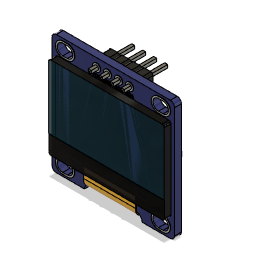
Tela OLed 128x64 v15 (Autodesk Fusion 360 design; units mm, degrees)
Autodesk Fusion 360 part; units mm, degrees
(part 1 of 2)
sketch "Sketch1" plane through (0, 0, 0) normal (0, 0, 1) x (1, 0, 0)
  line L0 (13.34, -9.6) -> (-13.34, -9.6)
  line L1 (-13.34, -9.6) -> (-13.34, 9.6)
  line L2 (-13.34, 9.6) -> (13.34, 9.6)
  line L3 (13.34, 9.6) -> (13.34, -9.6)
  line L4 (13.34, -9.6) -> (-13.34, 9.6) construction
  line L5 (-13.34, -9.6) -> (13.34, 9.6) construction
  dimension "d1" = 26.68
  dimension "d2" = 19.2
  constraint horizontal L0
  constraint perpendicular L0 L1
  constraint parallel L0 L2
  constraint parallel L1 L3
  constraint coincident L4 origin
  constraint coincident L5 origin
  measures "d1" distance of L1.end L2.end
  measures "d2" distance of L0.end L1.end
extrude "Extrude1" add sketch "Sketch1" along normal blind 1.5 makes body 1
sketch "Sketch2" plane through (0, 0, 1.5) normal (0, 0, 1) x (1, 0, 0)
  line L0 (13.34, 9.6) -> (-13.34, 9.6)
  line L1 (-13.34, 9.6) -> (-13.34, -9.6)
  line L2 (-13.34, -9.6) -> (13.34, -9.6)
  line L3 (13.34, -9.6) -> (13.34, 9.6)
  line L4 (-13.34, 9.6) -> (13.34, 9.6)
  line L5 (13.34, 9.6) -> (13.34, -5.4)
  line L6 (13.34, -5.4) -> (-13.34, -5.4)
  line L7 (-13.34, -5.4) -> (-13.34, 9.6)
  dimension "d5" = 15
  constraint horizontal L4
  constraint vertical L5
  constraint horizontal L6
  constraint vertical L7
  constraint coincident L3 L5.end
  constraint coincident L0.end L1.start
  measures "d5" distance of L0.end L6.end
extrude "Extrude2" add sketch "Sketch2" along normal blind 0.1 contours L0 L1 L3 L4 L5 L6 L7 bodies 1
copy_body "Body->Comp1" bodies 1 removing the originals makes body 2 in component "Pantalla"
sketch "Sketch1 (2)" plane through (0, 0, 0) normal (0, 0, -1) x (-1, 0, 0) in component "Base PCB"
  line L0 (13.34, 9.6) -> (-13.34, 9.6) construction
  line L1 (-13.34, 9.6) -> (-13.34, -9.6) construction
  line L2 (-13.34, -9.6) -> (13.34, -9.6) construction
  line L3 (13.34, -9.6) -> (13.34, 9.6) construction
  line L4 (-14.15, 14.25) -> (14.15, 14.25)
  line L5 (14.15, 14.25) -> (14.15, -13.4)
  line L6 (14.15, -13.4) -> (-14.15, -13.4)
  line L7 (-14.15, -13.4) -> (-14.15, 14.25)
  dimension "d8" = 27.65
  dimension "d9" = 28.3
  dimension "d10" = 3.8
  dimension "d11" = 0.81
  constraint horizontal L4
  constraint vertical L5
  constraint horizontal L6
  constraint vertical L7
  measures "d8" distance of L4.end L5.end
  measures "d9" distance of L4.start L4.end
  measures "d10" distance of L2 L6
  measures "d11" distance of L1 L7
extrude "Extrude1'" add sketch "Sketch1 (2)" along normal blind 1.6 separate body makes body 3 in component "Base PCB"
sketch "Sketch2 (2)" plane through (0, 0, 0) normal (0, 0, 1) x (1, 0, 0) in component "Base PCB"
  line L0 (-14.15, -13.4) -> (14.15, -13.4)
  line L1 (14.15, -13.4) -> (14.15, 14.25)
  line L2 (14.15, 14.25) -> (-14.15, 14.25)
  line L3 (-14.15, 14.25) -> (-14.15, -13.4)
  line L4 (-11.575, 10.9) -> (-10.525, 10.9) construction
  arc A0 (-10.525, 10.9) -> (-10.525, 13.25) centre (-10.525, 12.075) ccw construction
  line L5 (-10.525, 13.25) -> (-11.575, 13.25) construction
  arc A1 (-11.575, 13.25) -> (-11.575, 10.9) centre (-11.575, 12.075) ccw construction
  line L6 (-11.575, 12.075) -> (-10.525, 12.075) construction
  line L7 (0, 14.25) -> (0, 0) construction
  line L8 (0, 0) -> (14.15, 0) construction
  arc A2 (-10.525, 10.8) -> (-10.525, 13.35) centre (-10.525, 12.075) ccw
  line L9 (-10.525, 13.35) -> (-11.575, 13.35)
  arc A3 (-11.575, 13.35) -> (-11.575, 10.8) centre (-11.575, 12.075) ccw
  line L10 (-11.575, 10.8) -> (-10.525, 10.8)
  arc A4 (10.525, 13.35) -> (10.525, 10.8) centre (10.525, 12.075) ccw
  line L11 (10.525, 13.35) -> (11.575, 13.35)
  arc A5 (11.575, 10.8) -> (11.575, 13.35) centre (11.575, 12.075) ccw
  line L12 (11.575, 10.8) -> (10.525, 10.8)
  line L13 (-14.15, 0.425) -> (-23.1438, 0.425) construction
  line L14 (-10.525, -12.5) -> (-11.575, -12.5)
  arc A6 (-11.575, -9.95) -> (-11.575, -12.5) centre (-11.575, -11.225) ccw
  line L15 (-11.575, -9.95) -> (-10.525, -9.95)
  arc A7 (-10.525, -12.5) -> (-10.525, -9.95) centre (-10.525, -11.225) ccw
  line L16 (10.525, -12.5) -> (11.575, -12.5)
  arc A8 (10.525, -9.95) -> (10.525, -12.5) centre (10.525, -11.225) ccw
  line L17 (11.575, -9.95) -> (10.525, -9.95)
  arc A9 (11.575, -12.5) -> (11.575, -9.95) centre (11.575, -11.225) ccw
  point P0 (-12.75, 12.075)
  dimension "d14" = 1.175
  dimension "d15" = 1.05
  dimension "d16" = 1
  dimension "d17" = 1.4
  dimension "d18" = 0.1
  constraint tangent L4 A0
  constraint tangent A0 L5
  constraint parallel L4 L5
  constraint tangent L5 A1
  constraint tangent L4 A1
  constraint horizontal L6
  constraint midpoint A1 P0
  constraint midpoint L2 L7.start
  constraint coincident L7.end L8.start
  constraint coincident L1 L8.end
  constraint perpendicular L1 L8
  constraint symmetric L7 A2.end A4.start
  constraint symmetric L7 A2.start A4.end
  constraint symmetric L7 A2 A4
  constraint symmetric L7 L9.end L11.end
  constraint symmetric L7 A3.end A5.start
  constraint symmetric L7 A3 A5
  constraint midpoint L3 L13.start
  constraint perpendicular L3 L13
  constraint symmetric A2.end L13 L14.start
  constraint symmetric A2.start L13 L15.end
  constraint symmetric A2 L13 A7
  constraint symmetric L9.end L13 L14.end
  constraint symmetric A3.end L13 A6.start
  constraint symmetric A3 L13 A6
  constraint symmetric A4.end L13 A8.start
  constraint symmetric A4.start L13 L16.start
  constraint symmetric A4 L13 A8
  constraint symmetric L11.end L13 L16.end
  constraint symmetric A5.start L13 L17.start
  constraint symmetric A5 L13 A9
  measures "d14" radius of A1
  measures "d15" distance of A1.centre A0.centre
  measures "d16" distance of L2 L5
  measures "d17" distance of L3 P0
extrude "Extrude2'" cut sketch "Sketch2 (2)" against normal through all contours A2 L9 A3 L10 | A4 L11 A5 L12 | L14 A6 L15 A7 | L16 A8 L17 A9 bodies 3 in component "Base PCB"
fillet "Fillet1" radius 1 4 edges at (-14.15, 14.25, -0.8) (14.15, 14.25, -0.8) (-14.15, -13.4, -0.8) (14.15, -13.4, -0.8) on bodies 3 in component "Base PCB"
sketch "Sketch3" plane through (0, 0, 0) normal (0, 0, 1) x (1, 0, 0) in component "Base PCB"
  line L0 (10.525, 13.35) -> (11.575, 13.35)
  arc A0 (11.575, 10.8) -> (11.575, 13.35) centre (11.575, 12.075) ccw
  line L1 (11.575, 10.8) -> (10.525, 10.8)
  arc A1 (10.525, 13.35) -> (10.525, 10.8) centre (10.525, 12.075) ccw
  line L2 (-11.575, -9.95) -> (-10.525, -9.95)
  arc A2 (-10.525, -12.5) -> (-10.525, -9.95) centre (-10.525, -11.225) ccw
  line L3 (-10.525, -12.5) -> (-11.575, -12.5)
  arc A3 (-11.575, -9.95) -> (-11.575, -12.5) centre (-11.575, -11.225) ccw
  arc A4 (-11.575, 13.35) -> (-11.575, 10.8) centre (-11.575, 12.075) ccw
  line L4 (-11.575, 13.35) -> (-10.525, 13.35)
  arc A5 (-10.525, 10.8) -> (-10.525, 13.35) centre (-10.525, 12.075) ccw
  line L5 (-10.525, 10.8) -> (-11.575, 10.8)
  line L6 (11.575, -12.5) -> (10.525, -12.5)
  arc A6 (10.525, -9.95) -> (10.525, -12.5) centre (10.525, -11.225) ccw
  line L7 (10.525, -9.95) -> (11.575, -9.95)
  arc A7 (11.575, -12.5) -> (11.575, -9.95) centre (11.575, -11.225) ccw
  arc A8 (13.15, -13.4) -> (14.15, -12.4) centre (13.15, -12.4) ccw
  line L8 (14.15, -12.4) -> (14.15, 13.25)
  arc A9 (14.15, 13.25) -> (13.15, 14.25) centre (13.15, 13.25) ccw
  line L9 (13.15, 14.25) -> (-13.15, 14.25)
  arc A10 (-13.15, 14.25) -> (-14.15, 13.25) centre (-13.15, 13.25) ccw
  line L10 (-14.15, 13.25) -> (-14.15, -12.4)
  arc A11 (-14.15, -12.4) -> (-13.15, -13.4) centre (-13.15, -12.4) ccw
  line L11 (-13.15, -13.4) -> (13.15, -13.4)
  line L12 (-5.5683, 12.35) -> (5.9249, 12.35) construction
  circle A12 centre (-1.27, 12.35) radius 0.5
  circle A13 centre (-1.27, 12.35) radius 0.9
  line L13 (0, 14.25) -> (0, 16.388) construction
  circle A14 centre (-3.81, 12.35) radius 0.5
  circle A15 centre (-3.81, 12.35) radius 0.9
  circle A16 centre (3.81, 12.35) radius 0.9
  circle A17 centre (3.81, 12.35) radius 0.5
  circle A18 centre (1.27, 12.35) radius 0.9
  circle A19 centre (1.27, 12.35) radius 0.5
  dimension "d22" = 1.9
  dimension "d23" = 1
  dimension "d24" = 0.4
  dimension "d25" = 1.27
  dimension "d26" = 2.54
  constraint parallel L5 L12
  constraint coincident L12 A12.centre
  constraint midpoint L9 L13.start
  constraint perpendicular L9 L13
  constraint coincident L12 A14.centre
  constraint concentric A14 A15
  constraint equal A12 A14
  constraint equal A13 A15
  constraint symmetric A12 L13 A19
  constraint symmetric A13 L13 A18
  constraint symmetric L13 A14 A17
  constraint symmetric L13 A15 A16
  measures "d22" distance of L9 L12
  measures "d23" diameter of A12
  measures "d25" distance of A12.centre L13
  measures "d26" distance of A12.centre A14.centre
extrude "Extrude3" cut sketch "Sketch3" against normal through all contours A12 | A14 | A17 | A19 bodies 3 in component "Base PCB"
extrude "Extrude4" add sketch "Sketch3" along normal blind 0.1 contours A13 | A15 | A16 | A18 bodies 3 in component "Base PCB"
sketch "Sketch4" plane through (0, 0, 0) normal (0, 0, 1) x (1, 0, 0) in component "Base PCB"
  circle A0 centre (3.81, 12.35) radius 0.9
  circle A1 centre (-3.81, 12.35) radius 0.9
  circle A2 centre (1.27, 12.35) radius 0.9
  circle A3 centre (-1.27, 12.35) radius 0.9
  line L0 (10.525, 13.35) -> (11.575, 13.35)
  arc A4 (11.575, 10.8) -> (11.575, 13.35) centre (11.575, 12.075) ccw
  line L1 (11.575, 10.8) -> (10.525, 10.8)
  arc A5 (10.525, 13.35) -> (10.525, 10.8) centre (10.525, 12.075) ccw
  line L2 (-11.575, -9.95) -> (-10.525, -9.95)
  arc A6 (-10.525, -12.5) -> (-10.525, -9.95) centre (-10.525, -11.225) ccw
  line L3 (-10.525, -12.5) -> (-11.575, -12.5)
  arc A7 (-11.575, -9.95) -> (-11.575, -12.5) centre (-11.575, -11.225) ccw
  arc A8 (-11.575, 13.35) -> (-11.575, 10.8) centre (-11.575, 12.075) ccw
  line L4 (-11.575, 13.35) -> (-10.525, 13.35)
  arc A9 (-10.525, 10.8) -> (-10.525, 13.35) centre (-10.525, 12.075) ccw
  line L5 (-10.525, 10.8) -> (-11.575, 10.8)
  line L6 (11.575, -12.5) -> (10.525, -12.5)
  arc A10 (10.525, -9.95) -> (10.525, -12.5) centre (10.525, -11.225) ccw
  line L7 (10.525, -9.95) -> (11.575, -9.95)
  arc A11 (11.575, -12.5) -> (11.575, -9.95) centre (11.575, -11.225) ccw
  arc A12 (13.15, -13.4) -> (14.15, -12.4) centre (13.15, -12.4) ccw
  line L8 (14.15, -12.4) -> (14.15, 13.25)
  arc A13 (14.15, 13.25) -> (13.15, 14.25) centre (13.15, 13.25) ccw
  line L9 (13.15, 14.25) -> (-13.15, 14.25)
  arc A14 (-13.15, 14.25) -> (-14.15, 13.25) centre (-13.15, 13.25) ccw
  line L10 (-14.15, 13.25) -> (-14.15, -12.4)
  arc A15 (-14.15, -12.4) -> (-13.15, -13.4) centre (-13.15, -12.4) ccw
  line L11 (-13.15, -13.4) -> (13.15, -13.4)
  arc A16 (-10.525, 10.4) -> (-10.525, 13.75) centre (-10.525, 12.075) ccw
  line L12 (-11.575, 13.75) -> (-10.525, 13.75)
  arc A17 (-11.575, 13.75) -> (-11.575, 10.4) centre (-11.575, 12.075) ccw
  line L13 (-10.525, 10.4) -> (-11.575, 10.4)
  line L14 (10.525, 13.75) -> (11.575, 13.75)
  arc A18 (11.575, 10.4) -> (11.575, 13.75) centre (11.575, 12.075) ccw
  line L15 (11.575, 10.4) -> (10.525, 10.4)
  arc A19 (10.525, 13.75) -> (10.525, 10.4) centre (10.525, 12.075) ccw
  line L16 (-11.575, -9.55) -> (-10.525, -9.55)
  arc A20 (-10.525, -12.9) -> (-10.525, -9.55) centre (-10.525, -11.225) ccw
  line L17 (-10.525, -12.9) -> (-11.575, -12.9)
  arc A21 (-11.575, -9.55) -> (-11.575, -12.9) centre (-11.575, -11.225) ccw
  line L18 (10.525, -9.55) -> (11.575, -9.55)
  arc A22 (11.575, -12.9) -> (11.575, -9.55) centre (11.575, -11.225) ccw
  line L19 (11.575, -12.9) -> (10.525, -12.9)
  arc A23 (10.525, -9.55) -> (10.525, -12.9) centre (10.525, -11.225) ccw
  dimension "d30" = -0.4
  dimension "d31" = 0.4
  dimension "d32" = 0.4
  dimension "d33" = 0.4
extrude "Extrude5" add sketch "Sketch4" along normal blind 0.1 contours A16 L12 A17 L13 | L14 A18 L15 A19 | L16 A20 L17 A21 | L18 A22 L19 A23 bodies 3 in component "Base PCB"
sketch "Sketch5" plane through (0, 0, 0) normal (0, 0, 1) x (1, 0, 0) in component "Base PCB"
  line L0 (-11.575, 13.75) -> (-10.525, 13.75)
  arc A0 (-10.525, 10.4) -> (-10.525, 13.75) centre (-10.525, 12.075) ccw
  line L1 (-10.525, 10.4) -> (-11.575, 10.4)
  arc A1 (-11.575, 13.75) -> (-11.575, 10.4) centre (-11.575, 12.075) ccw
  line L2 (-10.525, -12.9) -> (-11.575, -12.9)
  arc A2 (-11.575, -9.55) -> (-11.575, -12.9) centre (-11.575, -11.225) ccw
  line L3 (-11.575, -9.55) -> (-10.525, -9.55)
  arc A3 (-10.525, -12.9) -> (-10.525, -9.55) centre (-10.525, -11.225) ccw
  line L4 (11.575, 10.4) -> (10.525, 10.4)
  arc A4 (10.525, 13.75) -> (10.525, 10.4) centre (10.525, 12.075) ccw
  line L5 (10.525, 13.75) -> (11.575, 13.75)
  arc A5 (11.575, 10.4) -> (11.575, 13.75) centre (11.575, 12.075) ccw
  line L6 (11.575, -12.9) -> (10.525, -12.9)
  arc A6 (10.525, -9.55) -> (10.525, -12.9) centre (10.525, -11.225) ccw
  line L7 (10.525, -9.55) -> (11.575, -9.55)
  arc A7 (11.575, -12.9) -> (11.575, -9.55) centre (11.575, -11.225) ccw
  circle A8 centre (3.81, 12.35) radius 0.9
  circle A9 centre (-3.81, 12.35) radius 0.9
  circle A10 centre (1.27, 12.35) radius 0.9
  circle A11 centre (-1.27, 12.35) radius 0.9
  arc A12 (13.15, -13.4) -> (14.15, -12.4) centre (13.15, -12.4) ccw
  line L8 (14.15, -12.4) -> (14.15, 13.25)
  arc A13 (14.15, 13.25) -> (13.15, 14.25) centre (13.15, 13.25) ccw
  line L9 (13.15, 14.25) -> (-13.15, 14.25)
  arc A14 (-13.15, 14.25) -> (-14.15, 13.25) centre (-13.15, 13.25) ccw
  line L10 (-14.15, 13.25) -> (-14.15, -12.4)
  arc A15 (-14.15, -12.4) -> (-13.15, -13.4) centre (-13.15, -12.4) ccw
  line L11 (-13.15, -13.4) -> (13.15, -13.4)
  line L12 (-5.1944, 10.2341) -> (-2.4915, 10.2341) construction
  line L13 (-2.4915, 10.2341) -> (-2.4915, 11.0501) construction
  line L14 (-2.4915, 11.0501) -> (-5.1944, 11.0501) construction
  line L15 (-5.1944, 11.0501) -> (-5.1944, 10.2341) construction
  line L16 (-2.6944, 10.2341) -> (0.0085, 10.2341) construction
  line L17 (0.0085, 10.2341) -> (0.0085, 11.0501) construction
  line L18 (0.0085, 11.0501) -> (-2.6944, 11.0501) construction
  line L19 (-2.6944, 11.0501) -> (-2.6944, 10.2341) construction
  line L20 (-0.0944, 10.2341) -> (2.6085, 10.2341) construction
  line L21 (2.6085, 10.2341) -> (2.6085, 11.0501) construction
  line L22 (2.6085, 11.0501) -> (-0.0944, 11.0501) construction
  line L23 (-0.0944, 11.0501) -> (-0.0944, 10.2341) construction
  line L24 (2.4056, 10.2341) -> (5.1085, 10.2341) construction
  line L25 (5.1085, 10.2341) -> (5.1085, 11.0501) construction
  line L26 (5.1085, 11.0501) -> (2.4056, 11.0501) construction
  line L27 (2.4056, 11.0501) -> (2.4056, 10.2341) construction
  dimension "d36" = 0.7
  dimension "d38" = 0.7
  dimension "d39" = 0.7
  dimension "d40" = 0.7
  text T0 "VCC" font "Arial" height 0.7 align centre top in box 2.7029 x 0.816 at (-5.1944, 10.2341) x (1, 0) y (0, 1) spacing 1 kerned
  text T1 "GND" font "Arial" height 0.7 align centre top in box 2.7029 x 0.816 at (-2.6944, 10.2341) x (1, 0) y (0, 1) spacing 1 kerned
  text T2 "SCL\n" font "Arial" height 0.7 align centre top in box 2.7029 x 0.816 at (-0.0944, 10.2341) x (1, 0) y (0, 1) spacing 1 kerned
  text T3 "SDA\n" font "Arial" height 0.7 align centre top in box 2.7029 x 0.816 at (2.4056, 10.2341) x (1, 0) y (0, 1) spacing 1 kerned
extrude "Extrude6" add sketch "Sketch5" along normal blind 0.1 text T0 T1 T2 T3 bodies 3 in component "Base PCB"
sketch "Sketch1 (3)" plane through (0, 0, 0.1) normal (0, 0, 1) x (1, 0, 0) in component "PINOS"
  circle A0 centre (-3.81, 12.35) radius 0.5
  circle A1 centre (-3.81, 12.35) radius 0.9
  line L0 (-3.46, 12) -> (-4.16, 12)
  line L1 (-4.16, 12) -> (-4.16, 12.7)
  line L2 (-4.16, 12.7) -> (-3.46, 12.7)
  line L3 (-3.46, 12.7) -> (-3.46, 12)
  line L4 (-3.46, 12) -> (-4.16, 12.7) construction
  line L5 (-4.16, 12) -> (-3.46, 12.7) construction
  point P0 (-3.81, 12.35)
  dimension "d43" = 0.7
  dimension "d44" = 0.7
  constraint horizontal L0
  constraint perpendicular L0 L1
  constraint parallel L0 L2
  constraint parallel L1 L3
  constraint coincident L4 P0
  constraint coincident L5 P0
  constraint coincident P0 A0.centre
  measures "d43" distance of L1.end L2.end
  measures "d44" distance of L0.end L1.end
extrude "Extrude1''" add sketch "Sketch1 (3)" along normal blind 1.7 and the other way blind 8.7 separate body contours L0 L1 L2 L3 makes body 4 in component "PINOS"
chamfer "Chamfer1" distance 0.2 angle 45 1 faces at (-3.6933, 12.2333, -8.6) on bodies 4 in component "PINOS"
sketch "Sketch2 (3)" plane through (0, 0, -8.6) normal (0, 0, -1) x (-1, 0, 0) in component "PINOS"
  line L0 (3.66, 12.2) -> (3.96, 12.2)
  line L1 (3.96, 12.2) -> (3.96, 12.5)
  line L2 (3.96, 12.5) -> (3.66, 12.5)
  line L3 (3.66, 12.5) -> (3.66, 12.2)
  line L4 (5.08, 11.08) -> (2.54, 11.08)
  line L5 (2.54, 11.08) -> (2.54, 13.62)
  line L6 (2.54, 13.62) -> (5.08, 13.62)
  line L7 (5.08, 13.62) -> (5.08, 11.08)
  line L8 (5.08, 11.08) -> (2.54, 13.62) construction
  line L9 (2.54, 11.08) -> (5.08, 13.62) construction
  point P0 (3.81, 12.35)
  dimension "d50" = 2.54
  dimension "d51" = 2.54
  constraint horizontal L4
  constraint perpendicular L4 L5
  constraint parallel L4 L6
  constraint parallel L5 L7
  constraint coincident L8 P0
  constraint coincident L9 P0
  measures "d50" distance of L5.end L6.end
  measures "d51" distance of L4.end L5.end
extrude "Extrude2''" add sketch "Sketch2 (3)" along normal blind 2.5 from surface at -7 bodies 4 in component "PINOS"
fillet "Fillet1'" radius 0.5 4 edges at (-2.54, 13.62, -2.85) (-2.54, 11.08, -2.85) (-5.08, 11.08, -2.85) (-5.08, 13.62, -2.85) on bodies 4 in component "PINOS"
chamfer "Chamfer2" distance 0.2 angle 45 1 faces at (-3.6933, 12.2333, 1.8) on bodies 4 in component "PINOS"
pattern_linear "R-Pattern1" count 4 spacing 2.54 along (1, 0, 0) of bodies 4 makes body 5 at (-1.3867, 13.3133, -1.6) makes body 6 at (1.1533, 13.3133, -1.6) makes body 7 at (3.6933, 13.3133, -1.6) in component "PINOS"
sketch "Sketch6" plane through (0, 0, 0) normal (0, 0, 1) x (1, 0, 0) in component "Base PCB"
  line L0 (2.773, 10.575) -> (2.8604, 10.5826)
  spline S0 degree 3 poles (2.8604, 10.5826) (2.8628, 10.5663) (2.8674, 10.5359) (2.8823, 10.509) (2.8892, 10.4964) knots 0 0 0 0 0.004891 0.009154 0.009154 0.009154 0.009154
  spline S1 degree 3 poles (2.8892, 10.4964) (2.8983, 10.4856) (2.9177, 10.4623) (2.9451, 10.449) (2.9597, 10.442) knots 0 0 0 0 0.004201 0.008993 0.008993 0.008993 0.008993
  spline S2 degree 3 poles (2.9597, 10.442) (2.9764, 10.4359) (3.0111, 10.4234) (3.048, 10.422) (3.0671, 10.4212) knots 0 0 0 0 0.005307 0.011001 0.011001 0.011001 0.011001
  spline S3 degree 3 poles (3.0671, 10.4212) (3.0839, 10.4217) (3.1158, 10.4227) (3.1463, 10.4324) (3.1607, 10.437) knots 0 0 0 0 0.005005 0.009531 0.009531 0.009531 0.009531
  spline S4 degree 3 poles (3.1607, 10.437) (3.1731, 10.4424) (3.1964, 10.4525) (3.2132, 10.4714) (3.2211, 10.4802) knots 0 0 0 0 0.004002 0.007505 0.007505 0.007505 0.007505
  spline S5 degree 3 poles (3.2211, 10.4802) (3.2269, 10.4895) (3.2383, 10.5079) (3.2401, 10.5295) (3.2409, 10.5401) knots 0 0 0 0 0.003233 0.006393 0.006393 0.006393 0.006393
  spline S6 degree 3 poles (3.2409, 10.5401) (3.2402, 10.5507) (3.2387, 10.5715) (3.2274, 10.589) (3.2218, 10.5977) knots 0 0 0 0 0.003123 0.006151 0.006151 0.006151 0.006151
  spline S7 degree 3 poles (3.2218, 10.5977) (3.2138, 10.6058) (3.1957, 10.6239) (3.1719, 10.6336) (3.1588, 10.639) knots 0 0 0 0 0.003394 0.007604 0.007604 0.007604 0.007604
  spline S8 degree 3 poles (3.1588, 10.639) (3.1438, 10.6438) (3.1027, 10.6569) (3.0607, 10.6668) (3.0342, 10.6731) knots 0 0 0 0 0.004737 0.012926 0.012926 0.012926 0.012926
  spline S9 degree 3 poles (3.0342, 10.6731) (3.0065, 10.6797) (2.9603, 10.6907) (2.9166, 10.7093) (2.899, 10.7168) knots 0 0 0 0 0.008504 0.014223 0.014223 0.014223 0.014223
  spline S10 degree 3 poles (2.899, 10.7168) (2.8836, 10.7257) (2.8544, 10.7426) (2.834, 10.7693) (2.8243, 10.782) knots 0 0 0 0 0.005272 0.010003 0.010003 0.010003 0.010003
  spline S11 degree 3 poles (2.8243, 10.782) (2.8171, 10.7954) (2.8026, 10.8227) (2.8007, 10.8535) (2.7997, 10.8691) knots 0 0 0 0 0.004518 0.009149 0.009149 0.009149 0.009149
  spline S12 degree 3 poles (2.7997, 10.8691) (2.801, 10.8866) (2.8037, 10.9218) (2.821, 10.9526) (2.8298, 10.9682) knots 0 0 0 0 0.005182 0.010468 0.010468 0.010468 0.010468
  spline S13 degree 3 poles (2.8298, 10.9682) (2.8413, 10.9828) (2.8651, 11.0129) (2.8997, 11.0295) (2.9177, 11.0381) knots 0 0 0 0 0.005488 0.011363 0.011363 0.011363 0.011363
  spline S14 degree 3 poles (2.9177, 11.0381) (2.9378, 11.0451) (2.9794, 11.0595) (3.0234, 11.0612) (3.0461, 11.062) knots 0 0 0 0 0.006357 0.013128 0.013128 0.013128 0.013128
  spline S15 degree 3 poles (3.0461, 11.062) (3.0708, 11.0612) (3.1178, 11.0596) (3.1622, 11.0443) (3.1834, 11.0369) knots 0 0 0 0 0.00735 0.014025 0.014025 0.014025 0.014025
  spline S16 degree 3 poles (3.1834, 11.0369) (3.2019, 11.0278) (3.238, 11.0101) (3.2628, 10.9785) (3.2748, 10.9632) knots 0 0 0 0 0.006103 0.011883 0.011883 0.011883 0.011883
  spline S17 degree 3 poles (3.2748, 10.9632) (3.2843, 10.9463) (3.3034, 10.9119) (3.3073, 10.8727) (3.3092, 10.8529) knots 0 0 0 0 0.005746 0.011664 0.011664 0.011664 0.011664
  line L1 (3.3092, 10.8529) -> (3.2204, 10.8462)
  spline S18 degree 3 poles (3.2204, 10.8462) (3.217, 10.8666) (3.2108, 10.9049) (3.1843, 10.9332) (3.1719, 10.9465) knots 0 0 0 0 0.006033 0.011362 0.011362 0.011362 0.011362
  spline S19 degree 3 poles (3.1719, 10.9465) (3.1553, 10.9563) (3.1179, 10.9785) (3.0742, 10.9797) (3.0499, 10.9804) knots 0 0 0 0 0.005712 0.012847 0.012847 0.012847 0.012847
  spline S20 degree 3 poles (3.0499, 10.9804) (3.0251, 10.98) (2.9816, 10.9793) (2.9437, 10.9585) (2.9274, 10.9496) knots 0 0 0 0 0.007305 0.012798 0.012798 0.012798 0.012798
  spline S21 degree 3 poles (2.9274, 10.9496) (2.9162, 10.9391) (2.8946, 10.9188) (2.8908, 10.8894) (2.889, 10.8753) knots 0 0 0 0 0.004455 0.008597 0.008597 0.008597 0.008597
  spline S22 degree 3 poles (2.889, 10.8753) (2.8901, 10.8633) (2.8923, 10.8396) (2.9083, 10.822) (2.9162, 10.8132) knots 0 0 0 0 0.003505 0.006945 0.006945 0.006945 0.006945
  spline S23 degree 3 poles (2.9162, 10.8132) (2.9321, 10.8044) (2.9757, 10.7801) (3.0247, 10.7699) (3.0559, 10.7633) knots 0 0 0 0 0.005421 0.014902 0.014902 0.014902 0.014902
  spline S24 degree 3 poles (3.0559, 10.7633) (3.0879, 10.7562) (3.1405, 10.7445) (3.191, 10.726) (3.2108, 10.7187) knots 0 0 0 0 0.009816 0.01614 0.01614 0.01614 0.01614
  spline S25 degree 3 poles (3.2108, 10.7187) (3.2295, 10.7092) (3.2644, 10.6915) (3.2894, 10.6614) (3.3011, 10.6473) knots 0 0 0 0 0.006198 0.011615 0.011615 0.011615 0.011615
  spline S26 degree 3 poles (3.3011, 10.6473) (3.3096, 10.6322) (3.3269, 10.6013) (3.3291, 10.5658) (3.3302, 10.5478) knots 0 0 0 0 0.005137 0.010493 0.010493 0.010493 0.010493
  spline S27 degree 3 poles (3.3302, 10.5478) (3.3288, 10.5293) (3.326, 10.4918) (3.3075, 10.4591) (3.2982, 10.4425) knots 0 0 0 0 0.005484 0.011123 0.011123 0.011123 0.011123
  spline S28 degree 3 poles (3.2982, 10.4425) (3.2861, 10.4268) (3.2611, 10.3944) (3.2249, 10.3754) (3.2063, 10.3656) knots 0 0 0 0 0.005873 0.012108 0.012108 0.012108 0.012108
  spline S29 degree 3 poles (3.2063, 10.3656) (3.1853, 10.3576) (3.1419, 10.341) (3.0954, 10.3391) (3.0714, 10.3381) knots 0 0 0 0 0.006693 0.013847 0.013847 0.013847 0.013847
  spline S30 degree 3 poles (3.0714, 10.3381) (3.042, 10.3389) (2.9875, 10.3403) (2.9359, 10.3578) (2.9122, 10.3658) knots 0 0 0 0 0.00876 0.016246 0.016246 0.016246 0.016246
  spline S31 degree 3 poles (2.9122, 10.3658) (2.892, 10.3761) (2.8522, 10.3964) (2.8249, 10.4317) (2.8114, 10.4492) knots 0 0 0 0 0.006698 0.01322 0.01322 0.01322 0.01322
  spline S32 degree 3 poles (2.8114, 10.4492) (2.8007, 10.4685) (2.7789, 10.5076) (2.775, 10.5523) (2.773, 10.575) knots 0 0 0 0 0.00655 0.013288 0.013288 0.013288 0.013288
  line L2 (-0.8872, 10.3501) -> (-0.8872, 11.0501)
  line L3 (-0.8872, 11.0501) -> (-0.646, 11.0501)
  spline S33 degree 3 poles (-0.646, 11.0501) (-0.622, 11.05) (-0.5801, 11.0498) (-0.5389, 11.043) (-0.5214, 11.0401) knots 0 0 0 0 0.007203 0.01252 0.01252 0.01252 0.01252
  spline S34 degree 3 poles (-0.5214, 11.0401) (-0.5023, 11.0347) (-0.465, 11.0242) (-0.4339, 11.0011) (-0.4187, 10.9899) knots 0 0 0 0 0.005905 0.01151 0.01151 0.01151 0.01151
  spline S35 degree 3 poles (-0.4187, 10.9899) (-0.4014, 10.973) (-0.3659, 10.9386) (-0.346, 10.8933) (-0.3359, 10.8703) knots 0 0 0 0 0.0072 0.014672 0.014672 0.014672 0.014672
  spline S36 degree 3 poles (-0.3359, 10.8703) (-0.3279, 10.8445) (-0.3111, 10.7903) (-0.3093, 10.7336) (-0.3084, 10.7039) knots 0 0 0 0 0.008068 0.016934 0.016934 0.016934 0.016934
  spline S37 degree 3 poles (-0.3084, 10.7039) (-0.309, 10.6787) (-0.3102, 10.6309) (-0.3216, 10.5845) (-0.3271, 10.5626) knots 0 0 0 0 0.007535 0.014294 0.014294 0.014294 0.014294
  spline S38 degree 3 poles (-0.3271, 10.5626) (-0.3333, 10.5434) (-0.3452, 10.5075) (-0.3654, 10.4755) (-0.3748, 10.4606) knots 0 0 0 0 0.006016 0.011295 0.011295 0.011295 0.011295
  spline S39 degree 3 poles (-0.3748, 10.4606) (-0.3845, 10.4481) (-0.4029, 10.4241) (-0.427, 10.4058) (-0.4385, 10.3971) knots 0 0 0 0 0.004722 0.009034 0.009034 0.009034 0.009034
  spline S40 degree 3 poles (-0.4385, 10.3971) (-0.451, 10.3898) (-0.4773, 10.3744) (-0.5067, 10.3663) (-0.5221, 10.362) knots 0 0 0 0 0.004328 0.009098 0.009098 0.009098 0.009098
  spline S41 degree 3 poles (-0.5221, 10.362) (-0.5396, 10.3585) (-0.5767, 10.3512) (-0.6145, 10.3505) (-0.6346, 10.3501) knots 0 0 0 0 0.005334 0.011328 0.011328 0.011328 0.011328
  line L4 (-0.6346, 10.3501) -> (-0.8872, 10.3501)
  line L5 (1.5285, 10.5955) -> (1.6212, 10.5721)
  spline S42 degree 3 poles (1.6212, 10.5721) (1.6103, 10.5369) (1.5896, 10.4702) (1.5399, 10.4212) (1.5164, 10.3981) knots 0 0 0 0 0.010852 0.020599 0.020599 0.020599 0.020599
  spline S43 degree 3 poles (1.5164, 10.3981) (1.4892, 10.3806) (1.4328, 10.3444) (1.3659, 10.3403) (1.3313, 10.3381) knots 0 0 0 0 0.009535 0.019739 0.019739 0.019739 0.019739
  spline S44 degree 3 poles (1.3313, 10.3381) (1.2965, 10.3394) (1.2317, 10.3417) (1.1739, 10.3708) (1.1473, 10.3842) knots 0 0 0 0 0.010325 0.019174 0.019174 0.019174 0.019174
  spline S45 degree 3 poles (1.1473, 10.3842) (1.1249, 10.4017) (1.0786, 10.4378) (1.0527, 10.4905) (1.0393, 10.5177) knots 0 0 0 0 0.008414 0.017361 0.017361 0.017361 0.017361
  spline S46 degree 3 poles (1.0393, 10.5177) (1.0286, 10.5476) (1.0067, 10.6082) (1.0038, 10.6727) (1.0023, 10.7053) knots 0 0 0 0 0.009476 0.019225 0.019225 0.019225 0.019225
  spline S47 degree 3 poles (1.0023, 10.7053) (1.0037, 10.7399) (1.0064, 10.806) (1.0319, 10.867) (1.0441, 10.8961) knots 0 0 0 0 0.010289 0.019668 0.019668 0.019668 0.019668
  spline S48 degree 3 poles (1.0441, 10.8961) (1.0594, 10.9215) (1.0896, 10.9718) (1.1387, 11.0039) (1.163, 11.0198) knots 0 0 0 0 0.00877 0.017356 0.017356 0.017356 0.017356
  spline S49 degree 3 poles (1.163, 11.0198) (1.1896, 11.0321) (1.2434, 11.0571) (1.3027, 11.0604) (1.3328, 11.062) knots 0 0 0 0 0.008697 0.017635 0.017635 0.017635 0.017635
  spline S50 degree 3 poles (1.3328, 11.062) (1.3658, 11.0602) (1.4292, 11.0567) (1.4835, 11.0241) (1.5094, 11.0085) knots 0 0 0 0 0.009761 0.018708 0.018708 0.018708 0.018708
  spline S51 degree 3 poles (1.5094, 11.0085) (1.5316, 10.9884) (1.5776, 10.9468) (1.5984, 10.8883) (1.6092, 10.8581) knots 0 0 0 0 0.00885 0.0183 0.0183 0.0183 0.0183
  line L6 (1.6092, 10.8581) -> (1.518, 10.8366)
  spline S52 degree 3 poles (1.518, 10.8366) (1.5098, 10.8598) (1.4946, 10.9023) (1.4622, 10.9336) (1.4474, 10.9479) knots 0 0 0 0 0.007245 0.013338 0.013338 0.013338 0.013338
  spline S53 degree 3 poles (1.4474, 10.9479) (1.4304, 10.9581) (1.3946, 10.9795) (1.3528, 10.9816) (1.3309, 10.9828) knots 0 0 0 0 0.005846 0.012327 0.012327 0.012327 0.012327
  spline S54 degree 3 poles (1.3309, 10.9828) (1.3056, 10.9815) (1.2575, 10.9791) (1.2158, 10.9554) (1.196, 10.9441) knots 0 0 0 0 0.00747 0.014208 0.014208 0.014208 0.014208
  spline S55 degree 3 poles (1.196, 10.9441) (1.1792, 10.93) (1.1454, 10.9016) (1.1284, 10.8608) (1.1198, 10.8402) knots 0 0 0 0 0.006466 0.013046 0.013046 0.013046 0.013046
  spline S56 degree 3 poles (1.1198, 10.8402) (1.1134, 10.8183) (1.1006, 10.7744) (1.0988, 10.7287) (1.0978, 10.7058) knots 0 0 0 0 0.006821 0.013665 0.013665 0.013665 0.013665
  spline S57 degree 3 poles (1.0978, 10.7058) (1.0987, 10.6777) (1.1002, 10.6245) (1.1163, 10.5738) (1.1239, 10.5499) knots 0 0 0 0 0.008387 0.015874 0.015874 0.015874 0.015874
  spline S58 degree 3 poles (1.1239, 10.5499) (1.1335, 10.5293) (1.1521, 10.4892) (1.1876, 10.4631) (1.2048, 10.4504) knots 0 0 0 0 0.006702 0.013015 0.013015 0.013015 0.013015
  spline S59 degree 3 poles (1.2048, 10.4504) (1.2235, 10.4407) (1.2608, 10.4215) (1.3027, 10.4188) (1.3237, 10.4174) knots 0 0 0 0 0.006229 0.012455 0.012455 0.012455 0.012455
  spline S60 degree 3 poles (1.3237, 10.4174) (1.3484, 10.4191) (1.3964, 10.4223) (1.4362, 10.4492) (1.4555, 10.4623) knots 0 0 0 0 0.007273 0.014147 0.014147 0.014147 0.014147
  spline S61 degree 3 poles (1.4555, 10.4623) (1.4722, 10.48) (1.5081, 10.5179) (1.5214, 10.5685) (1.5285, 10.5955) knots 0 0 0 0 0.00718 0.015411 0.015411 0.015411 0.015411
  line L7 (0.3453, 10.575) -> (0.4327, 10.5826)
  spline S62 degree 3 poles (0.4327, 10.5826) (0.4352, 10.5663) (0.4398, 10.5359) (0.4547, 10.509) (0.4616, 10.4964) knots 0 0 0 0 0.004891 0.009154 0.009154 0.009154 0.009154
  spline S63 degree 3 poles (0.4616, 10.4964) (0.4707, 10.4856) (0.4901, 10.4623) (0.5174, 10.449) (0.532, 10.442) knots 0 0 0 0 0.004201 0.008993 0.008993 0.008993 0.008993
  spline S64 degree 3 poles (0.532, 10.442) (0.5488, 10.4359) (0.5835, 10.4234) (0.6204, 10.422) (0.6395, 10.4212) knots 0 0 0 0 0.005307 0.011001 0.011001 0.011001 0.011001
  spline S65 degree 3 poles (0.6395, 10.4212) (0.6562, 10.4217) (0.6882, 10.4227) (0.7186, 10.4324) (0.733, 10.437) knots 0 0 0 0 0.005005 0.009531 0.009531 0.009531 0.009531
  spline S66 degree 3 poles (0.733, 10.437) (0.7454, 10.4424) (0.7687, 10.4525) (0.7856, 10.4714) (0.7934, 10.4802) knots 0 0 0 0 0.004002 0.007505 0.007505 0.007505 0.007505
  spline S67 degree 3 poles (0.7934, 10.4802) (0.7992, 10.4895) (0.8107, 10.5079) (0.8124, 10.5295) (0.8133, 10.5401) knots 0 0 0 0 0.003233 0.006393 0.006393 0.006393 0.006393
  spline S68 degree 3 poles (0.8133, 10.5401) (0.8125, 10.5507) (0.811, 10.5715) (0.7997, 10.589) (0.7942, 10.5977) knots 0 0 0 0 0.003123 0.006151 0.006151 0.006151 0.006151
  spline S69 degree 3 poles (0.7942, 10.5977) (0.7861, 10.6058) (0.7681, 10.6239) (0.7443, 10.6336) (0.7311, 10.639) knots 0 0 0 0 0.003394 0.007604 0.007604 0.007604 0.007604
  spline S70 degree 3 poles (0.7311, 10.639) (0.7161, 10.6438) (0.675, 10.6569) (0.6331, 10.6668) (0.6065, 10.6731) knots 0 0 0 0 0.004737 0.012926 0.012926 0.012926 0.012926
  spline S71 degree 3 poles (0.6065, 10.6731) (0.5789, 10.6797) (0.5326, 10.6907) (0.4889, 10.7093) (0.4714, 10.7168) knots 0 0 0 0 0.008504 0.014223 0.014223 0.014223 0.014223
  spline S72 degree 3 poles (0.4714, 10.7168) (0.456, 10.7257) (0.4268, 10.7426) (0.4063, 10.7693) (0.3966, 10.782) knots 0 0 0 0 0.005272 0.010003 0.010003 0.010003 0.010003
  spline S73 degree 3 poles (0.3966, 10.782) (0.3895, 10.7954) (0.375, 10.8227) (0.373, 10.8535) (0.3721, 10.8691) knots 0 0 0 0 0.004518 0.009149 0.009149 0.009149 0.009149
  spline S74 degree 3 poles (0.3721, 10.8691) (0.3734, 10.8866) (0.376, 10.9218) (0.3934, 10.9526) (0.4021, 10.9682) knots 0 0 0 0 0.005182 0.010468 0.010468 0.010468 0.010468
  spline S75 degree 3 poles (0.4021, 10.9682) (0.4136, 10.9828) (0.4374, 11.0129) (0.4721, 11.0295) (0.49, 11.0381) knots 0 0 0 0 0.005488 0.011363 0.011363 0.011363 0.011363
  spline S76 degree 3 poles (0.49, 11.0381) (0.5101, 11.0451) (0.5517, 11.0595) (0.5957, 11.0612) (0.6184, 11.062) knots 0 0 0 0 0.006357 0.013128 0.013128 0.013128 0.013128
  spline S77 degree 3 poles (0.6184, 11.062) (0.6431, 11.0612) (0.6901, 11.0596) (0.7346, 11.0443) (0.7557, 11.0369) knots 0 0 0 0 0.00735 0.014025 0.014025 0.014025 0.014025
  spline S78 degree 3 poles (0.7557, 11.0369) (0.7742, 11.0278) (0.8103, 11.0101) (0.8351, 10.9785) (0.8472, 10.9632) knots 0 0 0 0 0.006103 0.011883 0.011883 0.011883 0.011883
  spline S79 degree 3 poles (0.8472, 10.9632) (0.8566, 10.9463) (0.8758, 10.9119) (0.8796, 10.8727) (0.8815, 10.8529) knots 0 0 0 0 0.005746 0.011664 0.011664 0.011664 0.011664
  line L8 (0.8815, 10.8529) -> (0.7927, 10.8462)
  spline S80 degree 3 poles (0.7927, 10.8462) (0.7894, 10.8666) (0.7831, 10.9049) (0.7567, 10.9332) (0.7443, 10.9465) knots 0 0 0 0 0.006033 0.011362 0.011362 0.011362 0.011362
  spline S81 degree 3 poles (0.7443, 10.9465) (0.7276, 10.9563) (0.6902, 10.9785) (0.6465, 10.9797) (0.6223, 10.9804) knots 0 0 0 0 0.005712 0.012847 0.012847 0.012847 0.012847
  spline S82 degree 3 poles (0.6223, 10.9804) (0.5974, 10.98) (0.554, 10.9793) (0.5161, 10.9585) (0.4998, 10.9496) knots 0 0 0 0 0.007305 0.012798 0.012798 0.012798 0.012798
  spline S83 degree 3 poles (0.4998, 10.9496) (0.4886, 10.9391) (0.467, 10.9188) (0.4632, 10.8894) (0.4613, 10.8753) knots 0 0 0 0 0.004455 0.008597 0.008597 0.008597 0.008597
  spline S84 degree 3 poles (0.4613, 10.8753) (0.4624, 10.8633) (0.4646, 10.8396) (0.4806, 10.822) (0.4886, 10.8132) knots 0 0 0 0 0.003505 0.006945 0.006945 0.006945 0.006945
  spline S85 degree 3 poles (0.4886, 10.8132) (0.5044, 10.8044) (0.548, 10.7801) (0.597, 10.7699) (0.6282, 10.7633) knots 0 0 0 0 0.005421 0.014902 0.014902 0.014902 0.014902
  spline S86 degree 3 poles (0.6282, 10.7633) (0.6602, 10.7562) (0.7128, 10.7445) (0.7634, 10.726) (0.7832, 10.7187) knots 0 0 0 0 0.009816 0.01614 0.01614 0.01614 0.01614
  spline S87 degree 3 poles (0.7832, 10.7187) (0.8018, 10.7092) (0.8368, 10.6915) (0.8618, 10.6614) (0.8734, 10.6473) knots 0 0 0 0 0.006198 0.011615 0.011615 0.011615 0.011615
  spline S88 degree 3 poles (0.8734, 10.6473) (0.8819, 10.6322) (0.8993, 10.6013) (0.9014, 10.5658) (0.9025, 10.5478) knots 0 0 0 0 0.005137 0.010493 0.010493 0.010493 0.010493
  spline S89 degree 3 poles (0.9025, 10.5478) (0.9011, 10.5293) (0.8983, 10.4918) (0.8799, 10.4591) (0.8706, 10.4425) knots 0 0 0 0 0.005484 0.011123 0.011123 0.011123 0.011123
  spline S90 degree 3 poles (0.8706, 10.4425) (0.8584, 10.4268) (0.8335, 10.3944) (0.7973, 10.3754) (0.7786, 10.3656) knots 0 0 0 0 0.005873 0.012108 0.012108 0.012108 0.012108
  spline S91 degree 3 poles (0.7786, 10.3656) (0.7576, 10.3576) (0.7142, 10.341) (0.6678, 10.3391) (0.6437, 10.3381) knots 0 0 0 0 0.006693 0.013847 0.013847 0.013847 0.013847
  spline S92 degree 3 poles (0.6437, 10.3381) (0.6144, 10.3389) (0.5598, 10.3403) (0.5083, 10.3578) (0.4845, 10.3658) knots 0 0 0 0 0.008759 0.016246 0.016246 0.016246 0.016246
  spline S93 degree 3 poles (0.4845, 10.3658) (0.4643, 10.3761) (0.4245, 10.3964) (0.3972, 10.4317) (0.3838, 10.4492) knots 0 0 0 0 0.006698 0.01322 0.01322 0.01322 0.01322
  spline S94 degree 3 poles (0.3838, 10.4492) (0.373, 10.4685) (0.3512, 10.5076) (0.3473, 10.5523) (0.3453, 10.575) knots 0 0 0 0 0.00655 0.013288 0.013288 0.013288 0.013288
  arc A0 (13.15, -13.4) -> (14.15, -12.4) centre (13.15, -12.4) ccw
  line L9 (14.15, -12.4) -> (14.15, 13.25)
  arc A1 (14.15, 13.25) -> (13.15, 14.25) centre (13.15, 13.25) ccw
  line L10 (13.15, 14.25) -> (-13.15, 14.25)
  arc A2 (-13.15, 14.25) -> (-14.15, 13.25) centre (-13.15, 13.25) ccw
  line L11 (-14.15, 13.25) -> (-14.15, -12.4)
  arc A3 (-14.15, -12.4) -> (-13.15, -13.4) centre (-13.15, -12.4) ccw
  line L12 (-13.15, -13.4) -> (13.15, -13.4)
  circle A4 centre (-1.27, 12.35) radius 0.9
  circle A5 centre (1.27, 12.35) radius 0.9
  circle A6 centre (-3.81, 12.35) radius 0.9
  circle A7 centre (3.81, 12.35) radius 0.9
  line L13 (11.575, -12.9) -> (10.525, -12.9)
  arc A8 (10.525, -9.55) -> (10.525, -12.9) centre (10.525, -11.225) ccw
  line L14 (10.525, -9.55) -> (11.575, -9.55)
  arc A9 (11.575, -12.9) -> (11.575, -9.55) centre (11.575, -11.225) ccw
  line L15 (11.575, 10.4) -> (10.525, 10.4)
  arc A10 (10.525, 13.75) -> (10.525, 10.4) centre (10.525, 12.075) ccw
  line L16 (10.525, 13.75) -> (11.575, 13.75)
  arc A11 (11.575, 10.4) -> (11.575, 13.75) centre (11.575, 12.075) ccw
  line L17 (-10.525, -12.9) -> (-11.575, -12.9)
  arc A12 (-11.575, -9.55) -> (-11.575, -12.9) centre (-11.575, -11.225) ccw
  line L18 (-11.575, -9.55) -> (-10.525, -9.55)
  arc A13 (-10.525, -12.9) -> (-10.525, -9.55) centre (-10.525, -11.225) ccw
  line L19 (-11.575, 13.75) -> (-10.525, 13.75)
  arc A14 (-10.525, 10.4) -> (-10.525, 13.75) centre (-10.525, 12.075) ccw
  line L20 (-10.525, 10.4) -> (-11.575, 10.4)
  arc A15 (-11.575, 13.75) -> (-11.575, 10.4) centre (-11.575, 12.075) ccw
  line L21 (4.0861, 10.3501) -> (4.3549, 11.0501)
  line L22 (4.3549, 11.0501) -> (4.4547, 11.0501)
  line L23 (4.4547, 11.0501) -> (4.7412, 10.3501)
  line L24 (4.7412, 10.3501) -> (4.6357, 10.3501)
  line L25 (4.6357, 10.3501) -> (4.554, 10.5621)
  line L26 (4.554, 10.5621) -> (4.2613, 10.5621)
  line L27 (4.2613, 10.5621) -> (4.1844, 10.3501)
  line L28 (4.1844, 10.3501) -> (4.0861, 10.3501)
  line L29 (-4.5825, 10.3501) -> (-4.8538, 11.0501)
  line L30 (-4.8538, 11.0501) -> (-4.7535, 11.0501)
  line L31 (-4.7535, 11.0501) -> (-4.5716, 10.5416)
  spline S95 degree 3 poles (-4.5716, 10.5416) (-4.5646, 10.5219) (-4.5513, 10.484) (-4.5402, 10.4455) (-4.5348, 10.427) knots 0 0 0 0 0.006255 0.012037 0.012037 0.012037 0.012037
  spline S96 degree 3 poles (-4.5348, 10.427) (-4.5291, 10.4461) (-4.5178, 10.4847) (-4.504, 10.5225) (-4.4971, 10.5416) knots 0 0 0 0 0.005993 0.012067 0.012067 0.012067 0.012067
  line L32 (-4.4971, 10.5416) -> (-4.308, 11.0501)
  line L33 (-4.308, 11.0501) -> (-4.2134, 11.0501)
  line L34 (-4.2134, 11.0501) -> (-4.4875, 10.3501)
  line L35 (-4.4875, 10.3501) -> (-4.5825, 10.3501)
  line L36 (-3.6309, 10.5955) -> (-3.5383, 10.5721)
  spline S97 degree 3 poles (-3.5383, 10.5721) (-3.5492, 10.5369) (-3.5699, 10.4702) (-3.6196, 10.4212) (-3.6431, 10.3981) knots 0 0 0 0 0.010852 0.020599 0.020599 0.020599 0.020599
  spline S98 degree 3 poles (-3.6431, 10.3981) (-3.6703, 10.3806) (-3.7266, 10.3444) (-3.7935, 10.3403) (-3.8281, 10.3381) knots 0 0 0 0 0.009535 0.019739 0.019739 0.019739 0.019739
  spline S99 degree 3 poles (-3.8281, 10.3381) (-3.863, 10.3394) (-3.9278, 10.3417) (-3.9855, 10.3708) (-4.0122, 10.3842) knots 0 0 0 0 0.010325 0.019174 0.019174 0.019174 0.019174
  spline S100 degree 3 poles (-4.0122, 10.3842) (-4.0346, 10.4017) (-4.0808, 10.4378) (-4.1067, 10.4905) (-4.1201, 10.5177) knots 0 0 0 0 0.008414 0.017361 0.017361 0.017361 0.017361
  spline S101 degree 3 poles (-4.1201, 10.5177) (-4.1309, 10.5476) (-4.1528, 10.6082) (-4.1557, 10.6727) (-4.1571, 10.7053) knots 0 0 0 0 0.009476 0.019225 0.019225 0.019225 0.019225
  spline S102 degree 3 poles (-4.1571, 10.7053) (-4.1557, 10.7399) (-4.153, 10.806) (-4.1275, 10.867) (-4.1153, 10.8961) knots 0 0 0 0 0.010289 0.019668 0.019668 0.019668 0.019668
  spline S103 degree 3 poles (-4.1153, 10.8961) (-4.1001, 10.9215) (-4.0699, 10.9718) (-4.0207, 11.0039) (-3.9964, 11.0198) knots 0 0 0 0 0.00877 0.017356 0.017356 0.017356 0.017356
  spline S104 degree 3 poles (-3.9964, 11.0198) (-3.9699, 11.0321) (-3.916, 11.0571) (-3.8567, 11.0604) (-3.8267, 11.062) knots 0 0 0 0 0.008697 0.017635 0.017635 0.017635 0.017635
  spline S105 degree 3 poles (-3.8267, 11.062) (-3.7936, 11.0602) (-3.7303, 11.0567) (-3.676, 11.0241) (-3.65, 11.0085) knots 0 0 0 0 0.009761 0.018708 0.018708 0.018708 0.018708
  spline S106 degree 3 poles (-3.65, 11.0085) (-3.6278, 10.9884) (-3.5819, 10.9468) (-3.561, 10.8883) (-3.5502, 10.8581) knots 0 0 0 0 0.00885 0.0183 0.0183 0.0183 0.0183
  line L37 (-3.5502, 10.8581) -> (-3.6414, 10.8366)
  spline S107 degree 3 poles (-3.6414, 10.8366) (-3.6497, 10.8598) (-3.6649, 10.9023) (-3.6973, 10.9336) (-3.7121, 10.9479) knots 0 0 0 0 0.007245 0.013338 0.013338 0.013338 0.013338
  spline S108 degree 3 poles (-3.7121, 10.9479) (-3.7291, 10.9581) (-3.7649, 10.9795) (-3.8066, 10.9816) (-3.8286, 10.9828) knots 0 0 0 0 0.005846 0.012327 0.012327 0.012327 0.012327
  spline S109 degree 3 poles (-3.8286, 10.9828) (-3.8539, 10.9815) (-3.9019, 10.9791) (-3.9437, 10.9554) (-3.9635, 10.9441) knots 0 0 0 0 0.00747 0.014208 0.014208 0.014208 0.014208
  spline S110 degree 3 poles (-3.9635, 10.9441) (-3.9802, 10.93) (-4.014, 10.9016) (-4.0311, 10.8608) (-4.0396, 10.8402) knots 0 0 0 0 0.006466 0.013046 0.013046 0.013046 0.013046
  spline S111 degree 3 poles (-4.0396, 10.8402) (-4.046, 10.8183) (-4.0589, 10.7744) (-4.0607, 10.7287) (-4.0616, 10.7058) knots 0 0 0 0 0.006821 0.013665 0.013665 0.013665 0.013665
  spline S112 degree 3 poles (-4.0616, 10.7058) (-4.0608, 10.6777) (-4.0592, 10.6245) (-4.0432, 10.5738) (-4.0356, 10.5499) knots 0 0 0 0 0.008387 0.015874 0.015874 0.015874 0.015874
  spline S113 degree 3 poles (-4.0356, 10.5499) (-4.026, 10.5293) (-4.0074, 10.4892) (-3.9719, 10.4631) (-3.9546, 10.4504) knots 0 0 0 0 0.006702 0.013015 0.013015 0.013015 0.013015
  spline S114 degree 3 poles (-3.9546, 10.4504) (-3.936, 10.4407) (-3.8986, 10.4215) (-3.8567, 10.4188) (-3.8358, 10.4174) knots 0 0 0 0 0.006229 0.012455 0.012455 0.012455 0.012455
  spline S115 degree 3 poles (-3.8358, 10.4174) (-3.8111, 10.4191) (-3.7631, 10.4223) (-3.7233, 10.4492) (-3.704, 10.4623) knots 0 0 0 0 0.007273 0.014147 0.014147 0.014147 0.014147
  spline S116 degree 3 poles (-3.704, 10.4623) (-3.6873, 10.48) (-3.6514, 10.5179) (-3.638, 10.5685) (-3.6309, 10.5955) knots 0 0 0 0 0.00718 0.015411 0.015411 0.015411 0.015411
  line L38 (-2.9247, 10.5955) -> (-2.8321, 10.5721)
  spline S117 degree 3 poles (-2.8321, 10.5721) (-2.843, 10.5369) (-2.8637, 10.4702) (-2.9134, 10.4212) (-2.9369, 10.3981) knots 0 0 0 0 0.010852 0.020599 0.020599 0.020599 0.020599
  spline S118 degree 3 poles (-2.9369, 10.3981) (-2.9641, 10.3806) (-3.0204, 10.3444) (-3.0873, 10.3403) (-3.1219, 10.3381) knots 0 0 0 0 0.009535 0.019739 0.019739 0.019739 0.019739
  spline S119 degree 3 poles (-3.1219, 10.3381) (-3.1568, 10.3394) (-3.2216, 10.3417) (-3.2793, 10.3708) (-3.306, 10.3842) knots 0 0 0 0 0.010325 0.019174 0.019174 0.019174 0.019174
  spline S120 degree 3 poles (-3.306, 10.3842) (-3.3284, 10.4017) (-3.3746, 10.4378) (-3.4005, 10.4905) (-3.4139, 10.5177) knots 0 0 0 0 0.008414 0.017361 0.017361 0.017361 0.017361
  spline S121 degree 3 poles (-3.4139, 10.5177) (-3.4247, 10.5476) (-3.4466, 10.6082) (-3.4494, 10.6727) (-3.4509, 10.7053) knots 0 0 0 0 0.009476 0.019225 0.019225 0.019225 0.019225
  spline S122 degree 3 poles (-3.4509, 10.7053) (-3.4495, 10.7399) (-3.4468, 10.806) (-3.4213, 10.867) (-3.4091, 10.8961) knots 0 0 0 0 0.010289 0.019668 0.019668 0.019668 0.019668
  spline S123 degree 3 poles (-3.4091, 10.8961) (-3.3939, 10.9215) (-3.3637, 10.9718) (-3.3145, 11.0039) (-3.2902, 11.0198) knots 0 0 0 0 0.00877 0.017356 0.017356 0.017356 0.017356
  spline S124 degree 3 poles (-3.2902, 11.0198) (-3.2637, 11.0321) (-3.2098, 11.0571) (-3.1505, 11.0604) (-3.1205, 11.062) knots 0 0 0 0 0.008697 0.017635 0.017635 0.017635 0.017635
  spline S125 degree 3 poles (-3.1205, 11.062) (-3.0874, 11.0602) (-3.0241, 11.0567) (-2.9698, 11.0241) (-2.9438, 11.0085) knots 0 0 0 0 0.009761 0.018708 0.018708 0.018708 0.018708
  spline S126 degree 3 poles (-2.9438, 11.0085) (-2.9216, 10.9884) (-2.8757, 10.9468) (-2.8548, 10.8883) (-2.844, 10.8581) knots 0 0 0 0 0.00885 0.0183 0.0183 0.0183 0.0183
  line L39 (-2.844, 10.8581) -> (-2.9352, 10.8366)
  spline S127 degree 3 poles (-2.9352, 10.8366) (-2.9435, 10.8598) (-2.9587, 10.9023) (-2.9911, 10.9336) (-3.0059, 10.9479) knots 0 0 0 0 0.007245 0.013338 0.013338 0.013338 0.013338
  spline S128 degree 3 poles (-3.0059, 10.9479) (-3.0229, 10.9581) (-3.0587, 10.9795) (-3.1004, 10.9816) (-3.1224, 10.9828) knots 0 0 0 0 0.005846 0.012327 0.012327 0.012327 0.012327
  spline S129 degree 3 poles (-3.1224, 10.9828) (-3.1477, 10.9815) (-3.1957, 10.9791) (-3.2375, 10.9554) (-3.2573, 10.9441) knots 0 0 0 0 0.00747 0.014208 0.014208 0.014208 0.014208
  spline S130 degree 3 poles (-3.2573, 10.9441) (-3.274, 10.93) (-3.3078, 10.9016) (-3.3248, 10.8608) (-3.3334, 10.8402) knots 0 0 0 0 0.006466 0.013046 0.013046 0.013046 0.013046
  spline S131 degree 3 poles (-3.3334, 10.8402) (-3.3398, 10.8183) (-3.3527, 10.7744) (-3.3545, 10.7287) (-3.3554, 10.7058) knots 0 0 0 0 0.006821 0.013665 0.013665 0.013665 0.013665
  spline S132 degree 3 poles (-3.3554, 10.7058) (-3.3546, 10.6777) (-3.353, 10.6245) (-3.337, 10.5738) (-3.3294, 10.5499) knots 0 0 0 0 0.008387 0.015874 0.015874 0.015874 0.015874
  spline S133 degree 3 poles (-3.3294, 10.5499) (-3.3198, 10.5293) (-3.3012, 10.4892) (-3.2657, 10.4631) (-3.2484, 10.4504) knots 0 0 0 0 0.006702 0.013015 0.013015 0.013015 0.013015
  spline S134 degree 3 poles (-3.2484, 10.4504) (-3.2298, 10.4407) (-3.1924, 10.4215) (-3.1505, 10.4188) (-3.1295, 10.4174) knots 0 0 0 0 0.006229 0.012455 0.012455 0.012455 0.012455
  spline S135 degree 3 poles (-3.1295, 10.4174) (-3.1049, 10.4191) (-3.0569, 10.4223) (-3.0171, 10.4492) (-2.9978, 10.4623) knots 0 0 0 0 0.007273 0.014147 0.014147 0.014147 0.014147
  spline S136 degree 3 poles (-2.9978, 10.4623) (-2.981, 10.48) (-2.9452, 10.5179) (-2.9318, 10.5685) (-2.9247, 10.5955) knots 0 0 0 0 0.00718 0.015411 0.015411 0.015411 0.015411
  line L40 (-1.5943, 10.3501) -> (-1.5943, 11.0501)
  line L41 (-1.5943, 11.0501) -> (-1.4993, 11.0501)
  line L42 (-1.4993, 11.0501) -> (-1.1316, 10.5005)
  line L43 (-1.1316, 10.5005) -> (-1.1316, 11.0501)
  line L44 (-1.1316, 11.0501) -> (-1.0428, 11.0501)
  line L45 (-1.0428, 11.0501) -> (-1.0428, 10.3501)
  line L46 (-1.0428, 10.3501) -> (-1.1378, 10.3501)
  line L47 (-1.1378, 10.3501) -> (-1.5055, 10.9001)
  line L48 (-1.5055, 10.9001) -> (-1.5055, 10.3501)
  line L49 (-1.5055, 10.3501) -> (-1.5943, 10.3501)
  line L50 (-2.0264, 10.6246) -> (-2.0264, 10.7068)
  line L51 (-2.0264, 10.7068) -> (-1.7299, 10.7072)
  line L52 (-1.7299, 10.7072) -> (-1.7299, 10.4475)
  spline S137 degree 3 poles (-1.7299, 10.4475) (-1.7525, 10.4306) (-1.7963, 10.3979) (-1.8464, 10.3761) (-1.8708, 10.3656) knots 0 0 0 0 0.008417 0.016343 0.016343 0.016343 0.016343
  spline S138 degree 3 poles (-1.8708, 10.3656) (-1.8951, 10.3576) (-1.9435, 10.3416) (-1.9944, 10.3393) (-2.0198, 10.3381) knots 0 0 0 0 0.007636 0.015212 0.015212 0.015212 0.015212
  spline S139 degree 3 poles (-2.0198, 10.3381) (-2.053, 10.3398) (-2.1182, 10.3431) (-2.1779, 10.3694) (-2.2072, 10.3823) knots 0 0 0 0 0.009904 0.0194 0.0194 0.0194 0.0194
  spline S140 degree 3 poles (-2.2072, 10.3823) (-2.2335, 10.3986) (-2.286, 10.4312) (-2.3183, 10.4838) (-2.3344, 10.51) knots 0 0 0 0 0.009158 0.018254 0.018254 0.018254 0.018254
  spline S141 degree 3 poles (-2.3344, 10.51) (-2.347, 10.5391) (-2.3726, 10.5987) (-2.3758, 10.6635) (-2.3774, 10.6967) knots 0 0 0 0 0.009414 0.019297 0.019297 0.019297 0.019297
  spline S142 degree 3 poles (-2.3774, 10.6967) (-2.3757, 10.7301) (-2.3723, 10.7961) (-2.3471, 10.8572) (-2.3347, 10.8875) knots 0 0 0 0 0.009936 0.019676 0.019676 0.019676 0.019676
  spline S143 degree 3 poles (-2.3347, 10.8875) (-2.3191, 10.915) (-2.2887, 10.9688) (-2.237, 11.0025) (-2.2117, 11.019) knots 0 0 0 0 0.009312 0.018243 0.018243 0.018243 0.018243
  spline S144 degree 3 poles (-2.2117, 11.019) (-2.1834, 11.0316) (-2.1245, 11.0576) (-2.0602, 11.0605) (-2.0269, 11.062) knots 0 0 0 0 0.009213 0.019119 0.019119 0.019119 0.019119
  spline S145 degree 3 poles (-2.0269, 11.062) (-2.0026, 11.0611) (-1.9557, 11.0595) (-1.9111, 11.0446) (-1.8896, 11.0374) knots 0 0 0 0 0.007254 0.014011 0.014011 0.014011 0.014011
  spline S146 degree 3 poles (-1.8896, 11.0374) (-1.8706, 11.0288) (-1.834, 11.0122) (-1.8066, 10.9829) (-1.7934, 10.9689) knots 0 0 0 0 0.006214 0.011914 0.011914 0.011914 0.011914
  spline S147 degree 3 poles (-1.7934, 10.9689) (-1.7823, 10.9524) (-1.7585, 10.9171) (-1.7467, 10.8762) (-1.7404, 10.8543) knots 0 0 0 0 0.005919 0.012695 0.012695 0.012695 0.012695
  line L53 (-1.7404, 10.8543) -> (-1.824, 10.8314)
  spline S148 degree 3 poles (-1.824, 10.8314) (-1.8291, 10.8477) (-1.8385, 10.8774) (-1.8555, 10.9036) (-1.8631, 10.9154) knots 0 0 0 0 0.005091 0.009309 0.009309 0.009309 0.009309
  spline S149 degree 3 poles (-1.8631, 10.9154) (-1.8721, 10.9253) (-1.8911, 10.946) (-1.9166, 10.958) (-1.93, 10.9644) knots 0 0 0 0 0.003955 0.008356 0.008356 0.008356 0.008356
  spline S150 degree 3 poles (-1.93, 10.9644) (-1.9451, 10.9697) (-1.9763, 10.9808) (-2.0094, 10.9821) (-2.0264, 10.9828) knots 0 0 0 0 0.004787 0.009869 0.009869 0.009869 0.009869
  spline S151 degree 3 poles (-2.0264, 10.9828) (-2.0464, 10.9822) (-2.0839, 10.981) (-2.1195, 10.9691) (-2.1363, 10.9634) knots 0 0 0 0 0.005941 0.011206 0.011206 0.011206 0.011206
  spline S152 degree 3 poles (-2.1363, 10.9634) (-2.1507, 10.9567) (-2.1785, 10.9439) (-2.2005, 10.9227) (-2.211, 10.9126) knots 0 0 0 0 0.004745 0.009095 0.009095 0.009095 0.009095
  spline S153 degree 3 poles (-2.211, 10.9126) (-2.2199, 10.9019) (-2.2376, 10.8807) (-2.2493, 10.8557) (-2.2552, 10.8433) knots 0 0 0 0 0.00416 0.008242 0.008242 0.008242 0.008242
  spline S154 degree 3 poles (-2.2552, 10.8433) (-2.263, 10.821) (-2.2789, 10.7754) (-2.2809, 10.7271) (-2.2819, 10.7025) knots 0 0 0 0 0.007059 0.014407 0.014407 0.014407 0.014407
  spline S155 degree 3 poles (-2.2819, 10.7025) (-2.281, 10.6734) (-2.2793, 10.6193) (-2.2591, 10.5691) (-2.2497, 10.5459) knots 0 0 0 0 0.008633 0.016101 0.016101 0.016101 0.016101
  spline S156 degree 3 poles (-2.2497, 10.5459) (-2.2378, 10.5262) (-2.2142, 10.4873) (-2.1752, 10.4639) (-2.1558, 10.4523) knots 0 0 0 0 0.006768 0.013431 0.013431 0.013431 0.013431